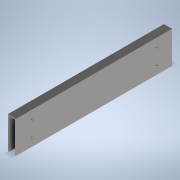
# Autodesk Inventor part: tankholder
Saved by Autodesk Inventor 2020 (Build 240168000, 168)
## iProperties
Created: 2020-07-20
Part Number: tankholder
Material: Generic
Document SubType Name: Modeling
Designer: Abbas
Density: 1 g/cm^3
Appearance: Default
Author: Abbas
Autodesk Inventor part; units mm, degrees
ref_plane "YZ Plane" through (0, 0, 0) normal (1, 0, 0) x (0, 1, 0)
ref_plane "XZ Plane" through (0, 0, 0) normal (0, 1, 0) x (-1, 0, 0)
ref_plane "XY Plane" through (0, 0, 0) normal (0, 0, 1) x (1, 0, 0)
sketch "Sketch1" plane through (0, 0, 0) normal (0, 0, 1) x (1, 0, 0)
  line L0 (-10, 50) -> (10, 50)
  line L1 (10, 50) -> (10, -50)
  line L2 (-10, -50) -> (-10, 50)
  line L3 (-10, 50) -> (10, -50) construction
  line L4 (10, 50) -> (-10, -50) construction
  line L5 (-13, 53) -> (13, 53)
  line L6 (13, 53) -> (13, -50)
  line L7 (-13, -50) -> (-13, 53)
  line L8 (-13, 53) -> (13, -53) construction
  line L9 (13, 53) -> (-13, -53) construction
  line L10 (-10, -50) -> (-13, -50)
  line L11 (10, -50) -> (13, -50)
  point P0 (0, 0)
  point P1 (0, 0)
  constraints: 24 end point, 5 midpoint, 4 perpendicular, 2 horizontal, 2 parallel
extrude "Extrusion1" add sketch "Sketch1" along normal blind 500
sketch "Sketch2" plane through (13, -50, 0) normal (1, 0, 0) x (0, 0, -1)
  line L0 (-500, 0) -> (-500, 103) projected
  line L1 (0, 0) -> (-500, 0) projected
  line L2 (0, 0) -> (0, 103) projected
  point P0 (0, 50)
  point P1 (-450, 75)
  point P2 (-450, 25)
  point P3 (-50, 75)
  point P4 (-50, 25)
  dimension "d21" = 50
  dimension "d22" = 50
  dimension "d23" = 50
  dimension "d24" = 25
  dimension "d25" = 50
  dimension "d26" = 25
  dimension "d27" = 50
  dimension "d28" = 50
  measures "d21" distance of point (-450, 25) point (-450, 75)
  measures "d22" distance from line of L0 point (-450, 25)
  measures "d23" distance from line of L0 point (-450, 75)
  measures "d24" distance from line of L1 point (-450, 25)
  measures "d25" distance of point (-50, 25) point (-50, 75)
  measures "d26" distance from line of L1 point (-50, 25)
  measures "d27" distance from line of L2 point (-50, 25)
  measures "d28" distance from line of L2 point (-50, 75)
hole "Hole1" at (13, 25, 450) at (13, -25, 450) at (13, 25, 50) at (13, -25, 50) direction (-1, 0, 0) diameter 6 end through all
body "Solid1"
